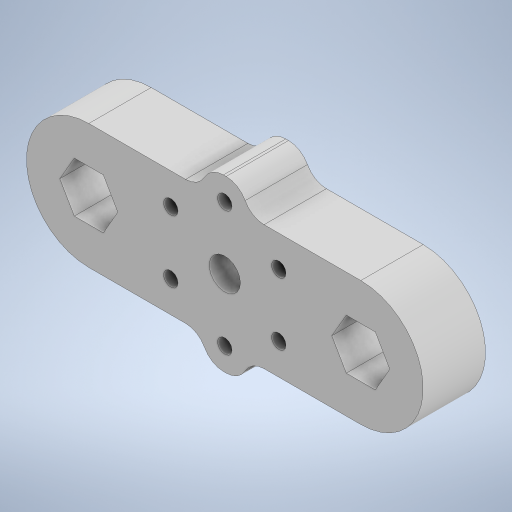
# Autodesk Inventor part: Part2
Saved by Autodesk Inventor 2024.2 (Build 282272000, 272)
## iProperties
Created: 2024-01-12
Part Number: Part2
Material: Generic
Document SubType Name: Modeling
Designer: AdminForWorker
Density: 1 g/cm^3
Appearance: Default
Author: AdminForWorker
Autodesk Inventor part; units mm, degrees
ref_plane "YZ Plane" through (0, 0, 0) normal (1, 0, 0) x (0, 1, 0)
ref_plane "XZ Plane" through (0, 0, 0) normal (0, 1, 0) x (-1, 0, 0)
ref_plane "XY Plane" through (0, 0, 0) normal (0, 0, 1) x (1, 0, 0)
sketch "Sketch7" plane through (0, 0, 0) normal (0, 0, 1) x (1, 0, 0)
  arc A0 (0, 16) -> (0, -16) centre (0, 0) ccw
  line L0 (0, 0) -> (4, 0)
  line L1 (0, 0) -> (7.448, 0)
  line L2 (7.448, 0) -> (11.448, 0)
  line L3 (62.36, 0) -> (69.808, 0)
  arc A1 (69.808, -16) -> (69.808, 16) centre (69.808, 0) ccw
  line L4 (7.448, 0) -> (3.724, 6.4502)
  line L5 (3.724, 6.4502) -> (-3.724, 6.4502)
  line L6 (-3.724, 6.4502) -> (-7.448, 0)
  line L7 (-7.448, 0) -> (-3.724, -6.4502)
  line L8 (-3.724, -6.4502) -> (3.724, -6.4502)
  line L9 (3.724, -6.4502) -> (7.448, 0)
  line L10 (62.36, 0) -> (66.084, 6.4502)
  line L11 (66.084, 6.4502) -> (73.532, 6.4502)
  line L12 (73.532, 6.4502) -> (77.256, 0)
  line L13 (77.256, 0) -> (73.532, -6.4502)
  line L14 (73.532, -6.4502) -> (66.084, -6.4502)
  line L15 (66.084, -6.4502) -> (62.36, 0)
  line L16 (64.7605, 16) -> (69.808, 16)
  line L17 (0, 16) -> (64.7605, 16)
  line L18 (0, 0) -> (34.904, 0)
  circle A2 centre (34.904, 0) radius 4
  line L19 (34.904, 0) -> (34.904, 16)
  circle A3 centre (34.904, 16) radius 1.85
  line L20 (34.904, 0) -> (34.904, -16)
  circle A4 centre (34.904, -16) radius 1.85
  line L21 (34.904, 0) -> (21.0475, 0)
  line L22 (21.0475, 0) -> (21.0475, -8)
  line L23 (21.0475, -8) -> (48.7605, -8)
  line L24 (48.7605, -8) -> (48.7605, 8)
  line L25 (48.7605, 8) -> (21.0475, 8)
  line L26 (21.0475, 8) -> (21.0475, 0)
  circle A5 centre (21.0475, 8) radius 1.85
  circle A6 centre (48.7605, 8) radius 1.85
  circle A7 centre (48.7605, -8) radius 1.85
  circle A8 centre (21.0475, -8) radius 1.85
  line L27 (34.904, -16) -> (34.904, -17.85)
  line L28 (34.904, -17.85) -> (34.904, -21.85)
  line L29 (34.904, 16) -> (34.904, 17.85)
  line L30 (34.904, 17.85) -> (34.904, 21.85)
  line L31 (34.904, -16) -> (33.054, -16)
  line L32 (29.0651, -16) -> (29.054, -16)
  line L33 (34.554, -21.85) -> (34.904, -21.85)
  line L34 (34.904, -16) -> (36.754, -16)
  line L35 (40.7429, -16) -> (40.754, -16)
  line L36 (35.254, -21.85) -> (34.904, -21.85)
  arc A9 (29.694, -18.925) -> (34.554, -21.85) centre (34.554, -16.35) ccw
  arc A10 (35.254, -21.85) -> (40.114, -18.925) centre (35.254, -16.35) ccw
  line L37 (0, -16) -> (24.834, -16)
  line L38 (33.054, -16) -> (36.754, -16)
  line L39 (44.974, -16) -> (69.808, -16)
  arc A11 (29.694, -18.925) -> (24.834, -16) centre (24.834, -21.5) ccw
  arc A12 (44.974, -16) -> (40.114, -18.925) centre (44.974, -21.5) ccw
  line L40 (34.904, 0) -> (34.904, 16)
  circle A13 centre (34.904, 16) radius 1.85
  line L41 (34.904, 16) -> (34.904, 17.85)
  line L42 (34.904, 17.85) -> (34.904, 21.85)
  line L43 (34.904, 16) -> (33.054, 16)
  line L44 (29.0651, 16) -> (29.054, 16)
  line L45 (34.554, 21.85) -> (34.904, 21.85)
  line L46 (34.904, 16) -> (36.754, 16)
  line L47 (40.7429, 16) -> (40.754, 16)
  line L48 (35.254, 21.85) -> (34.904, 21.85)
  arc A14 (34.554, 21.85) -> (29.694, 18.925) centre (34.554, 16.35) ccw
  arc A15 (40.114, 18.925) -> (35.254, 21.85) centre (35.254, 16.35) ccw
  line L49 (0, 16) -> (24.834, 16)
  line L50 (33.054, 16) -> (36.754, 16)
  line L51 (44.974, 16) -> (69.808, 16)
  arc A16 (24.834, 16) -> (29.694, 18.925) centre (24.834, 21.5) ccw
  arc A17 (40.114, 18.925) -> (44.974, 16) centre (44.974, 21.5) ccw
  point P0 (40.754, -21.85)
  point P1 (40.754, 21.85)
  dimension "d61" = 3.7
  dimension "d11" = 32
  dimension "d12" = 4
  dimension "d13" = 7.448
  dimension "d14" = 4
  dimension "d17" = 7.448
  dimension "d18" = 32
  dimension "d23" = 7.448
  dimension "d25" = 7.448
  dimension "d26" = 7.448
  dimension "d27" = 120
  dimension "d28" = 120
  dimension "d29" = 7.448
  dimension "d30" = 7.448
  dimension "d39" = 12.9003
  dimension "d41" = 12.9003
  dimension "d58" = 34.904
  dimension "d59" = 8
  dimension "d60" = 16
  dimension "d62" = 3.7
  dimension "d63" = 13.8565
  dimension "d64" = 8
  dimension "d65" = 27.713
  dimension "d66" = 16
  dimension "d67" = 27.713
  dimension "d68" = 90
  dimension "d69" = 3.7
  dimension "d70" = 3.7
  dimension "d71" = 3.7
  dimension "d72" = 3.7
  dimension "d73" = 4
  dimension "d74" = 4
  dimension "d77" = 5.5
  dimension "d78" = 5.5
  dimension "d79" = 5.5
  dimension "d80" = 5.5
  constraints: 104 end point, 32 point on circle, 23 symmetric about line, 17 centre point, 17 point on line, 13 tangent, 10 coincident, 7 parallel, 4 perpendicular, 3 horizontal, 2 midpoint, 2 vertical, 1 collinear, 1 vertical alignment, 7 other
  measures "d11" diameter of A0
  measures "d12" distance of L0.start L0.end
  measures "d13" distance of L0.start L1.end
  measures "d14" distance of L1.end L2.end
  measures "d17" distance of L3.start L3.end
  measures "d18" diameter of A1
  measures "d23" distance of L1.end L4.end
  measures "d25" distance of L4.end L5.end
  measures "d26" distance of L5.end L6.end
  measures "d27" angle of L6 L5
  measures "d28" angle of L7 L6
  measures "d29" distance of L7.end L8.end
  measures "d30" distance of L10.end L11.end
  measures "d39" distance between parallel lines of L12 L15
  measures "d41" distance between parallel lines of L13 L10
  measures "d58" distance of L0.start L18.end
  measures "d59" diameter of A2
  measures "d60" distance of L19.start L19.end
  measures "d62" diameter of A4
  measures "d63" distance of L19.start L21.end
  measures "d64" distance of L21.end L22.end
  measures "d65" distance of L22.end L23.end
  measures "d66" distance of L23.end L24.end
  measures "d67" distance of L24.end L25.end
  measures "d68" angle of L25 L24
  measures "d69" diameter of A5
  measures "d70" diameter of A6
  measures "d71" diameter of A7
  measures "d72" diameter of A8
  measures "d73" distance of L28.start L28.end
  measures "d74" distance of L29.end L30.end
  measures "d77" radius of A9
  measures "d78" radius of A10
  measures "d79" radius of A11
  measures "d80" radius of A12
extrude "Extrusion1" add sketch "Sketch7" along normal blind 16 contours L17 A3 L19 L25 A5 L26 L22 A8 L23 L20 A4 L28 L33 A9 A11 L37 A0 | A16 A14 L45 L30 A3 L17 | L48 A15 A17 L17 A3 L30 | L28 A4 L20 L23 A7 L24 A6 L25 L19 A3 L17 L16 A1 L39 A12 A10 L36 | L25 A6 L24 A7 L23 L20 A2 L19 | L19 A2 L18 L26 A5 L25 | A2 L20 L23 A8 L22 L18
body "Solid2"
